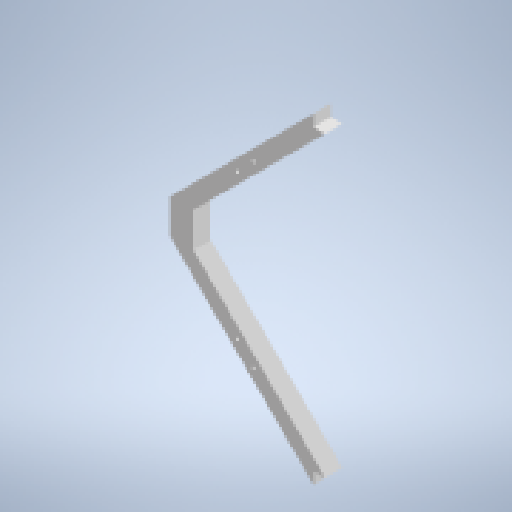
# Autodesk Inventor part: DOF6
Saved by Autodesk Inventor 2024 (Build 280153000, 153)
## iProperties
Created: 2024-10-16
Part Number: DOF6
Material: 一般
Document SubType Name: Modeling
Designer: jerry
Density: 1 g/cm^3
Appearance: 預設
Author: jerry
Autodesk Inventor part; units mm, degrees
ref_plane "YZ Plane" through (0, 0, 0) normal (1, 0, 0) x (0, 1, 0)
ref_plane "XZ Plane" through (0, 0, 0) normal (0, 1, 0) x (-1, 0, 0)
ref_plane "XY Plane" through (0, 0, 0) normal (0, 0, 1) x (1, 0, 0)
sketch "草圖1" plane through (0, 0, 0) normal (0, 0, 1) x (1, 0, 0)
  line L0 (165, 0) -> (165, -30)
  line L1 (165, 0) -> (195, 0) construction
  line L2 (165, -30) -> (391.2742, -256.2742)
  line L3 (391.2742, -256.2742) -> (371.2742, -256.2742)
  line L4 (371.2742, -256.2742) -> (371.2742, -276.2742)
  line L5 (371.2742, -276.2742) -> (123.7868, -28.7868)
  line L6 (165, 0) -> (165, 30)
  line L7 (165, 0) -> (195, 0) construction
  line L8 (165, 30) -> (391.2742, 256.2742)
  line L9 (391.2742, 256.2742) -> (371.2742, 256.2742)
  line L10 (371.2742, 256.2742) -> (371.2742, 276.2742)
  line L11 (371.2742, 276.2742) -> (123.7868, 28.7868)
  line L12 (123.7868, 28.7868) -> (123.7868, -28.7868)
  point P0 (0, 0)
  dimension "d3" = 30
  dimension "d4" = 90
  dimension "d5" = 320
  dimension "d6" = 135
  dimension "d7" = 20
  dimension "d8" = 20
  dimension "d9" = 350
  dimension "d10" = 45
  dimension "d11" = 30
  dimension "d12" = 90
  dimension "d13" = 320
  dimension "d14" = 135
  dimension "d15" = 20
  dimension "d16" = 20
  dimension "d17" = 350
  constraints: 26 end point, 6 perpendicular, 2 horizontal, 2 parallel, 1 vertical
  measures "d3" distance of L0.start L0.end
  measures "d4" angle of L0 L1
  measures "d5" distance of L0.end L2.end
  measures "d6" angle of L2 L0
  measures "d7" distance of L2.end L3.end
  measures "d8" distance of L3.end L4.end
  measures "d9" distance of L4.end L5.end
  measures "d10" angle of L4 L5
  measures "d11" distance of L0.start L6.end
  measures "d12" angle of L7 L6
  measures "d13" distance of L6.end L8.end
  measures "d14" angle of L6 L8
  measures "d15" distance of L8.end L9.end
  measures "d16" distance of L9.end L10.end
  measures "d17" distance of L10.end L11.end
extrude "擠出1" add sketch "草圖1" against normal blind 30
sketch "草圖2" plane through (0, 0, 0) normal (0, 0, 1) x (1, 0, 0)
  line L0 (391.2742, -256.2742) -> (371.2742, -256.2742) projected
  line L1 (371.2742, -256.2742) -> (315, -200)
  line L2 (371.2742, -256.2742) -> (450.8579, -256.2742) construction
  line L3 (315, -200) -> (290, -175)
  line L4 (123.7868, -28.7868) -> (371.2742, -276.2742) projected
  circle A0 centre (315, -200) radius 3
  circle A1 centre (290, -175) radius 3
  line L5 (371.2742, 256.2742) -> (391.2742, 256.2742) projected
  line L6 (371.2742, 256.2742) -> (315, 200)
  line L7 (371.2742, 276.2742) -> (123.7868, 28.7868) projected
  line L8 (371.2742, 256.2742) -> (450.8579, 256.2742) construction
  line L9 (315, 200) -> (290, 175)
  circle A2 centre (290, 175) radius 3
  circle A3 centre (315, 200) radius 3
  line L10 (315, -200) -> (315, 200)
  line L11 (290, -175) -> (290, 175)
  point P0 (0, 0)
  point P1 (317.1213, 202.1213)
  point P2 (312.8787, 197.8787)
  point P3 (312.8787, -197.8787)
  point P4 (317.1213, -202.1213)
  dimension "d20" = 79.5837
  dimension "d21" = 135
  dimension "d22" = 35.3553
  dimension "d23" = 180
  dimension "d24" = 6
  dimension "d25" = 6
  dimension "d28" = 79.5837
  dimension "d29" = 135
  dimension "d30" = 35.3553
  dimension "d31" = 6
  dimension "d32" = 6
  dimension "d33" = 400
  dimension "d34" = 350
  constraints: 16 end point, 4 centre point, 4 coincident, 2 equal length, 2 horizontal, 2 parallel, 1 point on line
  measures "d20" distance of L0.end L1.end
  measures "d21" angle of L2 L1
  measures "d22" distance of L1.end L3.end
  measures "d23" angle of L3 L1
  measures "d24" diameter of A0
  measures "d25" diameter of A1
  measures "d28" distance of L5.start L6.end
  measures "d29" angle of L6 L8
  measures "d30" distance of L6.end L9.end
  measures "d31" diameter of A2
  measures "d32" diameter of A3
  measures "d33" distance of L10.start L10.end
  measures "d34" distance of L11.start L11.end
extrude "擠出2" cut sketch "草圖2" along normal through all both and the other way through all contours A0 L3 L1 | L1 L10 A0 | L3 A0 L10 | A1 L11 L3 | L3 L11 A1 | L10 L6 A3 | A3 L9 L10 | A3 L6 L9 | L11 L9 A2 | A2 L9 L11
